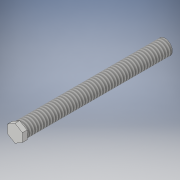
# Autodesk Inventor part: Pedal Bolt
Saved by Autodesk Inventor 2019 (Build 230136000, 136)
## iProperties
Created: 2020-06-01
Part Number: Pedal Bolt
Material: Generic
Document SubType Name: Modeling
Designer: 18186
Density: 1 g/cm^3
Appearance: Default
Author: 18186
Autodesk Inventor part; units mm, degrees
ref_plane "YZ Plane" through (0, 0, 0) normal (1, 0, 0) x (0, 1, 0)
ref_plane "XZ Plane" through (0, 0, 0) normal (0, 1, 0) x (-1, 0, 0)
ref_plane "XY Plane" through (0, 0, 0) normal (0, 0, 1) x (1, 0, 0)
sketch "Sketch1" plane through (0, 0, 0) normal (0, 0, 1) x (1, 0, 0)
  circle A0 centre (0, 0) radius 3.175
  dimension "d0" = 6.35
  constraints: 1 centre point, 1 coincident
  measures "d0" diameter of A0
extrude "Extrusion1" add sketch "Sketch1" along normal blind 62.4586
thread "Thread1" size "1/4-20 UNC" class "2A" standard "ANSI Unified Screw Threads" full length
sketch "Sketch2" plane through (0, 0, 62.4586) normal (0, 0, 1) x (1, 0, 0)
  line L0 (0, 3.683) -> (3.1896, 1.8415)
  line L1 (3.1896, 1.8415) -> (3.1896, -1.8415)
  line L2 (3.1896, -1.8415) -> (0, -3.683)
  line L3 (0, -3.683) -> (-3.1896, -1.8415)
  line L4 (-3.1896, -1.8415) -> (-3.1896, 1.8415)
  line L5 (-3.1896, 1.8415) -> (0, 3.683)
  point P0 (0, 0)
  point P1 (0, 0)
  dimension "d5" = 7.366
  constraints: 12 end point, 1 coincident, 13 other
  measures "d5" distance of L2.end L0.start
extrude "Extrusion2" add sketch "Sketch2" along normal blind 2
body "Solid1"
